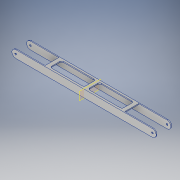
# Autodesk Inventor part: ArmProto2.2Assembly
Saved by Autodesk Inventor 2017 (Build 210142000, 142)
## iProperties
Created: 2017-10-04
Part Number: ArmProto2.2Assembly
Material: Aluminum 6061
Document SubType Name: Modeling
Designer: User
Density: 2.7 g/cm^3
Appearance: Aluminum - Flat
Mass: 245.529 g
Surface Area: 650.625 cm^2
Volume: 90.9365 cm^3
Author: User
Autodesk Inventor part; units mm, degrees
ref_plane "XZ Plane" through (0, 0, 0) normal (0, 1, 0) x (-1, 0, 0)
ref_plane "XY Plane" through (0, 0, 0) normal (0, 0, 1) x (1, 0, 0)
sketch "Sketch1" plane through (0, 0, 0) normal (1, 0, 0) x (0, 1, 0)
  line L0 (0, 0) -> (25.4, 0)
  line L1 (25.4, 0) -> (25.4, -52.3367)
  line L2 (25.4, -52.3367) -> (0, -52.3367)
  line L3 (0, -52.3367) -> (0, 0)
  line L4 (0, -3.175) -> (22.225, -3.175)
  line L5 (22.225, -3.175) -> (22.225, -49.1617)
  line L6 (22.225, -49.1617) -> (0, -49.1617)
  line L7 (0, -49.1617) -> (0, -3.175)
  dimension "d0" = 25.4
  dimension "d2" = 45.9867
  dimension "d3" = 22.225
  dimension "d4" = 3.175
  dimension "d32" = 3.175
  constraints: 16 end point, 4 parallel, 2 horizontal, 2 perpendicular, 1 point on line
  measures "d0" distance of L1.end L2.end
  measures "d2" distance of L4.end L5.end
  measures "d3" distance of L5.end L6.end
  measures "d4" distance between parallel lines of L0 L4
  measures "d32" distance between parallel lines of L6 L2
extrude "Extrusion1" add sketch "Sketch1" along normal blind 482.6 contours L0 L1 L2 L3 L6 L5 L4
sketch "Sketch3" plane through (0, 25.4, 0) normal (0, 1, 0) x (1, 0, 0)
  line L0 (0, 52.3367) -> (0, 0) projected
  line L1 (0, 0) -> (482.6, 0) projected
  line L2 (482.6, 52.3367) -> (482.6, 0) projected
  line L3 (0, 52.3367) -> (482.6, 52.3367) projected
  line L4 (482.6, 3.175) -> (374.65, 3.175)
  line L5 (374.65, 3.175) -> (374.65, 49.1617)
  line L6 (374.65, 49.1617) -> (482.6, 49.1617)
  line L7 (482.6, 49.1617) -> (482.6, 3.175)
  line L8 (0, 52.3367) -> (0, 0) projected
  line L9 (0, 3.175) -> (107.95, 3.175)
  line L10 (107.95, 3.175) -> (107.95, 49.1617)
  line L11 (107.95, 49.1617) -> (0, 49.1617)
  line L12 (0, 49.1617) -> (0, 3.175)
  point P0 (482.6, 49.1617)
  dimension "d14" = 52.3367
  dimension "d16" = 107.95
  dimension "d27" = 107.95
  dimension "d28" = 45.9867
  dimension "d29" = 3.175
  dimension "d30" = 45.9867
  dimension "d31" = 3.175
  constraints: 16 end point, 4 parallel, 2 horizontal, 2 perpendicular, 2 point on line
  measures "d14" distance of L0.start L0.end
  measures "d16" distance of L5.end L6.end
  measures "d27" distance of L11.end L10.end
  measures "d28" distance of L9.end L10.end
  measures "d29" distance between parallel lines of L3 L11
  measures "d30" distance of L4.end L5.end
  measures "d31" distance between parallel lines of L3 L6
extrude "Extrusion2" cut sketch "Sketch3" against normal blind 3.175 contours L11 L10 L9 L0 | L2 L4 L5 L6
fillet "Fillet1" radius 12.7 8 edges at (482.6, 25.4, -1.5875) (482.6, 0, -1.5875) (482.6, 25.4, -50.7492) (482.6, 0, -50.7492) (0, 25.4, -1.5875) (0, 0, -1.5875) (0, 0, -50.7492) (0, 25.4, -50.7492)
sketch "Sketch6" plane through (107.95, 25.4, -3.175) normal (0, 1, 0) x (1, 0, 0)
  line L0 (-95.25, 45.9867) -> (-95.25, 49.1617) projected
  line L1 (-95.25, 45.9867) -> (0, 45.9867) projected
  line L2 (0, 45.9867) -> (0, 0) projected
  line L3 (0, 0) -> (-95.25, 0) projected
  line L4 (-95.25, -3.175) -> (-95.25, 0) projected
  line L5 (-95.25, -3.175) -> (361.95, -3.175) projected
  line L6 (361.95, 0) -> (361.95, -3.175) projected
  line L7 (361.95, 0) -> (266.7, 0) projected
  line L8 (266.7, 0) -> (266.7, 45.9867) projected
  line L9 (266.7, 45.9867) -> (361.95, 45.9867) projected
  line L10 (361.95, 49.1617) -> (361.95, 45.9867) projected
  line L11 (-95.25, 49.1617) -> (361.95, 49.1617) projected
  line L12 (12.7, 42.8117) -> (127, 42.8117)
  line L13 (127, 42.8117) -> (127, 3.175)
  line L14 (127, 3.175) -> (12.7, 3.175)
  line L15 (12.7, 3.175) -> (12.7, 42.8117)
  point P0 (-107.95, -3.175)
  dimension "d65" = 266.7
  dimension "d66" = 52.3367
  dimension "d67" = 6.35
  dimension "d68" = 39.6367
  dimension "d69" = 12.7
  dimension "d70" = 114.3
  constraints: 8 end point, 2 parallel, 1 horizontal, 1 perpendicular
  measures "d65" distance between parallel lines of L8 L2
  measures "d66" distance between parallel lines of L5 L11
  measures "d67" distance between parallel lines of L11 L12
  measures "d68" distance of L14.end L12.start
  measures "d69" distance between parallel lines of L2 L15
  measures "d70" distance of L12.start L12.end
extrude "Extrusion4" cut sketch "Sketch6" against normal blind 25.4 contours L12 L13 L14 L15
fillet "Fillet2" radius 6.35 4 edges at (234.95, 23.8125, -45.9867) (234.95, 23.8125, -6.35) (120.65, 23.8125, -6.35) (120.65, 23.8125, -45.9867)
ref_plane "Work Plane1" through (241.3, 25.4, -52.3367) normal (1, 0, 0) x (0, 1, 0)
mirror "Mirror1" about plane through (241.3, 25.4, -52.3367) normal (1, 0, 0) of "Extrusion4"
fillet "Fillet3" radius 6.35 4 edges at (247.65, 23.8125, -6.35) (247.65, 23.8125, -45.9867) (361.95, 23.8125, -45.9867) (361.95, 23.8125, -6.35)
sketch "Sketch8" plane through (12.7, 0, 0) normal (0, 0, 1) x (1, 0, 0)
  arc A0 (0, 25.4) -> (0, 0) centre (0, 12.7) ccw projected
  line L0 (0, 0) -> (457.2, 0) projected
  arc A1 (457.2, 0) -> (457.2, 25.4) centre (457.2, 12.7) ccw projected
  line L1 (0, 25.4) -> (457.2, 25.4) projected
  line L2 (-2.5, 14.1435) -> (2.5, 14.1435)
  line L3 (2.5, 14.1435) -> (2.5, 11.2565)
  line L4 (2.5, 11.2565) -> (-2.5, 11.2565)
  line L5 (-2.5, 11.2565) -> (-2.5, 14.1435)
  line L6 (-2.5, 14.1435) -> (0, 15.5869)
  line L7 (-2.5, 14.1435) -> (1.2199, 14.1435) construction
  line L8 (2.5, 14.1435) -> (0, 15.5869)
  line L9 (2.5, 14.1435) -> (6.8654, 14.1435) construction
  line L10 (-2.5, 11.2565) -> (0, 9.8131)
  line L11 (-2.5, 11.2565) -> (2.5, 11.2565) construction
  line L12 (2.5, 11.2565) -> (0, 9.8131)
  line L13 (2.5, 11.2565) -> (7.3282, 11.2565) construction
  line L14 (2.5, 11.2565) -> (0, 9.8131)
  point P0 (-12.7, 0)
  dimension "d82" = 5
  dimension "d83" = 2.887
  dimension "d84" = 30
  dimension "d85" = 150
  dimension "d86" = 30
  dimension "d87" = 150
  dimension "d88" = 1.4435
  dimension "d89" = 2.5
  constraints: 26 end point, 5 horizontal, 3 equal length, 1 perpendicular
  measures "d82" distance of L3.end L4.end
  measures "d83" distance of L2.end L3.end
  measures "d84" angle of L7 L6
  measures "d85" angle of L9 L8
  measures "d86" angle of L10 L11
  measures "d87" angle of L12 L13
  measures "d88" distance from line of A0.centre L2
  measures "d89" distance from line of A0.centre L5
extrude "Extrusion5" cut sketch "Sketch8" against normal blind 76.2 contours L6 L8 L2 | L2 L3 L4 L5 | L4 L12 L10
mirror "Mirror2" about plane through (241.3, 25.4, -52.3367) normal (1, 0, 0) of "Extrusion5"
equation "\"d32\" = d4"
equation "\"d16\" = d27"
equation "\"d30\" = d28"
equation "\"d31\" = d29"
equation "\"d88\" = 0.5 * d83"
equation "\"d89\" = 0.5 * d82"
body "Solid1"
